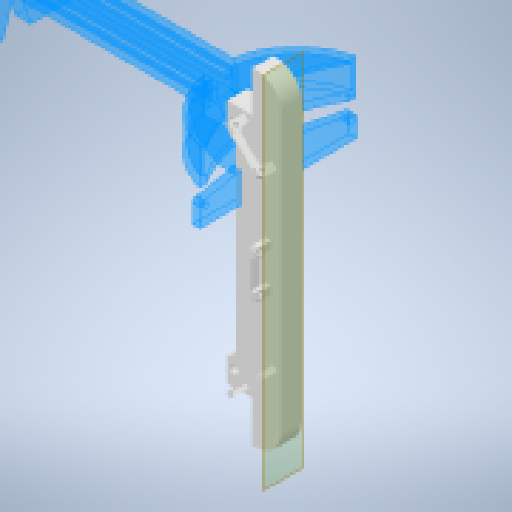
# Autodesk Inventor part: front_part_2
Saved by Autodesk Inventor 2023 (Build 270158000, 158)
## iProperties
Created: 2026-02-12
Part Number: front_part_2
Material: Типовые
Document SubType Name: Modeling
Designer: garin
Density: 1 g/cm^3
Appearance: По умолчанию
Author: garin
Autodesk Inventor part; units mm, degrees
ref_plane "YZ Plane" through (0, 0, 0) normal (1, 0, 0) x (0, 1, 0)
ref_plane "XZ Plane" through (0, 0, 0) normal (0, 1, 0) x (-1, 0, 0)
ref_plane "XY Plane" through (0, 0, 0) normal (0, 0, 1) x (1, 0, 0)
sketch "Эскиз1" plane through (0, 0, 0) normal (0, 0, 1) x (1, 0, 0)
  line L0 (0, 0) -> (90, 0)
  line L1 (90, 0) -> (90, 74.5)
  line L2 (123.0872, 0) -> (-138.0608, 0) construction
  line L3 (75, 74.5) -> (75, 65.5)
  line L4 (75, 65.5) -> (61.2, 65.5)
  line L5 (61.2, 65.5) -> (61.2, 52.2)
  line L6 (61.2, 52.2) -> (66.2, 52.2) construction
  line L7 (66.2, 52.2) -> (66.2, 47.2) construction
  line L8 (66.2, 47.2) -> (61.2, 47.2) construction
  line L9 (61.2, 47.2) -> (61.2, 52.2) construction
  arc A0 (66.2, 47.2) -> (61.2, 52.2) centre (61.2, 47.2) ccw
  line L10 (66.2, 47.2) -> (66.2, 0)
  line L11 (61.2, 52.2) -> (65.2, 52.2) construction
  line L12 (65.2, 52.2) -> (65.2, 57.2) construction
  line L13 (65.2, 57.2) -> (61.2, 57.2) construction
  line L14 (61.2, 57.2) -> (61.2, 52.2) construction
  circle A1 centre (65.2, 57.2) radius 2.1
  line L15 (75, 74.5) -> (75, 87.5)
  line L16 (75, 87.5) -> (77, 87.5)
  arc A2 (90, 74.5) -> (77, 87.5) centre (77, 74.5) ccw
  line L17 (90, 0) -> (90, -74.5)
  line L18 (75, -74.5) -> (75, -65.5)
  line L19 (75, -65.5) -> (61.2, -65.5)
  line L20 (61.2, -65.5) -> (61.2, -52.2)
  line L21 (61.2, -52.2) -> (66.2, -52.2) construction
  line L22 (66.2, -52.2) -> (66.2, -47.2) construction
  line L23 (66.2, -47.2) -> (61.2, -47.2) construction
  line L24 (61.2, -47.2) -> (61.2, -52.2) construction
  arc A3 (61.2, -52.2) -> (66.2, -47.2) centre (61.2, -47.2) ccw
  line L25 (66.2, -47.2) -> (66.2, 0)
  line L26 (61.2, -52.2) -> (65.2, -52.2) construction
  line L27 (65.2, -52.2) -> (65.2, -57.2) construction
  line L28 (65.2, -57.2) -> (61.2, -57.2) construction
  line L29 (61.2, -57.2) -> (61.2, -52.2) construction
  circle A4 centre (65.2, -57.2) radius 2.1
  line L30 (75, -74.5) -> (75, -87.5)
  line L31 (75, -87.5) -> (77, -87.5)
  arc A5 (77, -87.5) -> (90, -74.5) centre (77, -74.5) ccw
  circle A6 centre (81.192, 68.692) radius 2.1
  circle A7 centre (81.192, -68.692) radius 2.1
  line L32 (75, -65.5) -> (75, -37.341) construction
  line L33 (75, -37.341) -> (37.7624, -37.341) construction
  line L34 (66.2, -37.341) -> (74.621, -37.341) construction
  circle A8 centre (74.621, -37.341) radius 2.1
  circle A9 centre (74.621, 37.341) radius 2.1
  dimension "d0" = 90
  dimension "d1" = 74.5
  dimension "d2" = 15
  dimension "d3" = 9
  dimension "d4" = 13.8
  dimension "d5" = 13.3
  dimension "d6" = 5
  dimension "d7" = 5
  dimension "d8" = 4
  dimension "d9" = 5
  dimension "d10" = 4.2
  dimension "d13" = 13
  dimension "d14" = 2
  dimension "d49" = 4.2
  dimension "d83" = 28.159
  dimension "d84" = 8.421
  dimension "d85" = 4.2
  constraints: 70 end point, 18 symmetric about line, 10 centre point, 8 point on circle, 6 point on line, 5 perpendicular, 5 vertical, 4 horizontal, 4 parallel, 3 coincident, 2 tangent, 5 other
  measures "d0" distance of L0.start L0.end
  measures "d1" distance of L0.end L1.end
  measures "d2" distance of L1.end L3.start
  measures "d3" distance of L3.start L3.end
  measures "d4" distance of L3.end L4.end
  measures "d5" distance of L4.end L5.end
  measures "d6" distance of L7.end L8.end
  measures "d7" distance of L6.end L7.end
  measures "d8" distance of L13.end L12.end
  measures "d9" distance of L12.end L11.end
  measures "d10" diameter of A1
  measures "d13" distance of L3.start L15.end
  measures "d14" distance of L15.end L16.end
  measures "d49" diameter of A6
  measures "d83" distance of L19.start L32.end
  measures "d84" distance of L34.start L34.end
  measures "d85" diameter of A8
ref_plane "РабПлоскость1" through (-0.0152, -0.1454, 9) normal (0, 0, 1) x (0.9999948, 0.0032337, 0)
extrude "Выдавливание2" add sketch "Эскиз1" along normal blind 11 from surface at 9 contours L10 A0 L5 L4 L3 L15 L16 A2 L1 L0 | L0 L17 A5 L31 L30 L18 L19 L20 A3 L25 | A6 | A7 | A8 | A9
sketch "Эскиз2" plane through (61.2, -65.5, 20) normal (0, 0, 1) x (1, 0, 0)
  line L0 (0, 131) -> (13.8, 131) construction
  line L1 (0, 131) -> (7, 131) construction
  line L2 (7, 131) -> (7, 119) construction
  line L3 (7, 119) -> (0, 119) construction
  line L4 (0, 119) -> (0, 131) construction
  line L5 (7, 131) -> (7, 128) construction
  line L6 (26.9404, 112.3022) -> (24.8191, 110.1809)
  line L7 (24.8191, 110.1809) -> (7.1414, 127.8586)
  line L8 (24.8191, 110.1809) -> (49.8191, 110.1809) construction
  line L9 (7.1414, 127.8586) -> (9.2627, 129.9799)
  line L10 (9.2627, 129.9799) -> (26.9404, 112.3022)
  point P0 (-61.2, 65.5)
  dimension "d17" = 7
  dimension "d18" = 12
  dimension "d19" = 3
  dimension "d20" = 25.2
  dimension "d26" = 25
  dimension "d27" = 135
  constraints: 20 end point, 3 perpendicular, 2 horizontal, 2 parallel, 1 equal length, 1 point on line
  measures "d17" distance of L2.end L3.end
  measures "d18" distance of L1.end L2.end
  measures "d19" distance of L1.end L5.end
  measures "d20" distance of L5.end L6.end
  measures "d26" distance of L6.end L7.end
  measures "d27" angle of L8 L7
extrude "Выдавливание3" add sketch "Эскиз2" along normal blind 8.5
sketch "Эскиз4" plane through (70.4627, 64.4799, 20) normal (0.7071068, 0.7071068, 0) x (-0.7071068, 0.7071068, 0)
  line L0 (-25, 0) -> (-25, 8.5) construction
  line L1 (-25, 8.5) -> (-22.5, 8.5) construction
  line L2 (-25, 6) -> (-25, 8.5) construction
  circle A0 centre (-22.2, 6) radius 1.25
  circle A1 centre (-2.8, 6) radius 1.25
  line L3 (0, 8.5) -> (-25, 8.5) construction
  line L4 (-25, 8.5) -> (-21, 8.5) construction
  line L5 (-21, 8.5) -> (-21, 4.5) construction
  line L6 (-21, 4.5) -> (-25, 4.5) construction
  line L7 (-25, 4.5) -> (-25, 8.5) construction
  line L8 (-21, 4.5) -> (-4, 4.5)
  line L9 (-4, 4.5) -> (-4, 0)
  line L10 (-4, 0) -> (-21, 0)
  line L11 (-21, 0) -> (-21, 4.5)
  line L12 (-12.5, 8.5) -> (-12.5, 0) construction
  line L13 (-6.7296, 0) -> (-112.0886, 0) construction
  point P0 (4.2305, -20)
  point P1 (-22.5, 6)
  point P2 (-2.5, 6)
  point P3 (-2.8, 6)
  dimension "d31" = 2.5
  dimension "d32" = 2.5
  dimension "d33" = 4
  dimension "d34" = 4
  dimension "d35" = 17
  dimension "d36" = 4.5
  constraints: 22 end point, 4 parallel, 3 horizontal, 3 perpendicular, 2 centre point, 1 midpoint, 1 point on line
  measures "d31" diameter of A0
  measures "d32" diameter of A1
  measures "d33" distance of L5.end L6.end
  measures "d34" distance of L4.end L5.end
  measures "d35" distance of L9.end L10.end
  measures "d36" distance of L8.end L9.end
extrude "Выдавливание4" cut sketch "Эскиз4" against normal blind 3
fillet "Сопряжение1" radius 2 2 edges at (87.0798, 45.7416, 28.5) (69.4021, 63.4192, 28.5)
sketch "Эскиз6" plane through (71.1698, 59.5302, 24.5) normal (-0.7071068, -0.7071068, 0) x (-0.7071068, 0.7071068, 0)
  line L0 (-1, 0.0575) -> (-16, 0.0575)
  line L1 (-16, 0.0575) -> (-16, -4)
  line L2 (-16, -4) -> (-1, -4)
  line L3 (-1, -4) -> (-1, 0.0575)
  point P0 (8.2305, 24.5)
  dimension "d42" = 15
  constraints: 8 end point, 2 parallel, 1 horizontal, 1 perpendicular
  measures "d42" distance of L2.end L1.end
extrude "Выдавливание5" cut sketch "Эскиз6" along normal blind 2 from surface at -3
mirror "Зеркальное отражение1" about plane through (0, 0, 0) normal (0, 1, 0) of "Сопряжение1", "Выдавливание3", "Выдавливание4", "Выдавливание5"
extrude "Выдавливание6" cut sketch "Эскиз1" along normal blind 8 from surface at 9 contours A6 | A7
sketch "Эскиз8" plane through (61.2, 65.5, 20) normal (0, 0, 1) x (1, 0, 0)
  line L0 (28.8, 9) -> (28.8, -140) projected
  line L1 (23.8, -53) -> (20.8, -53)
  line L2 (20.8, -53) -> (20.8, -78)
  line L3 (20.8, -78) -> (23.8, -78)
  line L4 (23.8, -78) -> (23.8, -53)
  point P0 (-61.2, -65.5)
  point P1 (28.8, -63)
  point P2 (28.8, -65.5)
  dimension "d54" = 3
  dimension "d55" = 25
  constraints: 8 end point, 2 parallel, 1 horizontal, 1 midpoint, 1 perpendicular, 1 point on line
  measures "d54" distance of L3.end L2.end
  measures "d55" distance of L2.end L1.end
extrude "Выдавливание7" add sketch "Эскиз8" along normal blind 8.5
sketch "Эскиз10" plane through (85, -12.5, 20) normal (1, 0, 0) x (0, 0, -1)
  line L0 (-8.5, 25) -> (-8.5, 0) projected
  line L1 (-8.5, 0) -> (-6, 0) construction
  line L2 (-6, 0) -> (-6, 2.8) construction
  line L3 (-6, 2.8) -> (-8.5, 2.8) construction
  line L4 (-8.5, 2.8) -> (-8.5, 0) construction
  circle A0 centre (-6, 2.8) radius 1.25
  line L5 (-6, 2.8) -> (-6, 22.2) construction
  circle A1 centre (-6, 22.2) radius 1.25
  line L6 (-8.5, 0) -> (-4.5, 0) construction
  line L7 (-4.5, 0) -> (-4.5, 4) construction
  line L8 (-4.5, 4) -> (-8.5, 4) construction
  line L9 (-8.5, 4) -> (-8.5, 0) construction
  line L10 (-4.5, 4) -> (0, 4)
  line L11 (0, 4) -> (0, 21)
  line L12 (0, 21) -> (-4.5, 21)
  line L13 (-4.5, 21) -> (-4.5, 4)
  line L14 (-8.5, 0) -> (-8.5, 25) construction
  line L15 (-8.5, 0) -> (-8.5, 5) construction
  line L16 (-8.5, 5) -> (-4.5, 5)
  line L17 (-4.5, 5) -> (-4.5, 20)
  line L18 (-4.5, 20) -> (-8.5, 20)
  line L19 (-8.5, 20) -> (-8.5, 5)
  point P0 (20, 12.5)
  point P1 (-4.5, 5)
  dimension "d67" = 2.5
  dimension "d68" = 2.8
  dimension "d69" = 2.5
  dimension "d70" = 19.4
  dimension "d71" = 2.5
  dimension "d72" = 4
  dimension "d73" = 4
  dimension "d74" = 4.5
  dimension "d75" = 17
  dimension "d76" = 5
  dimension "d77" = 15
  constraints: 36 end point, 8 parallel, 4 horizontal, 4 perpendicular, 2 centre point, 2 coincident, 2 point on line, 1 vertical
  measures "d67" distance of L3.end L2.end
  measures "d68" distance of L2.end L1.end
  measures "d69" diameter of A0
  measures "d70" distance of L5.start L5.end
  measures "d71" diameter of A1
  measures "d72" distance of L8.end L7.end
  measures "d73" distance of L7.end L6.end
  measures "d74" distance of L12.end L11.end
  measures "d75" distance of L11.end L10.end
  measures "d76" distance of L0.end L15.end
  measures "d77" distance of L17.end L16.end
extrude "Выдавливание8" cut sketch "Эскиз10" against normal blind 3 contours L13 L12 L11 L10 | A0 | A1
extrude "Выдавливание9" cut sketch "Эскиз10" against normal blind 2 contours L18 L13 L16 L0
fillet "Сопряжение2" radius 2 2 edges at (83.5, 12.5, 28.5) (83.5, -12.5, 28.5)
ref_plane "РабПлоскость2" through (90, -37.25, 9) normal (-1, 0, 0) x (0, -1, 0)
extrude "Выдавливание10" cut sketch "Эскиз1" against normal blind 7 from surface at 20 contours A8 | A9
